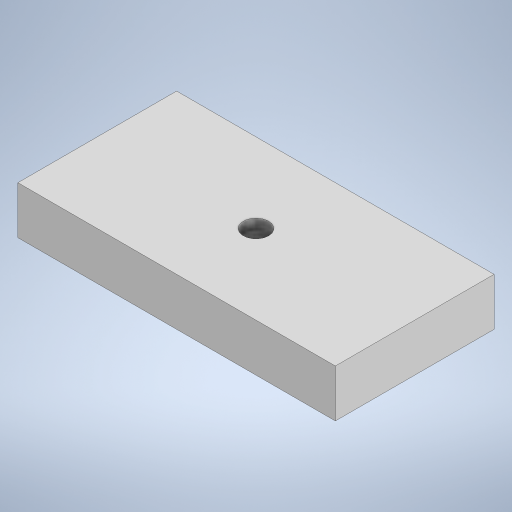
# Autodesk Inventor part: mocowanie osi
Saved by Autodesk Inventor 2024 (Build 280153000, 153)
## iProperties
Created: 2024-11-28
Part Number: mocowanie osi
Material: Ogólny
Document SubType Name: Modeling
Designer: fkoba.i_ekonomik
Density: 1 g/cm^3
Appearance: Domyślna
Author: fkoba.i_ekonomik
Autodesk Inventor part; units mm, degrees
ref_plane "YZ Plane" through (0, 0, 0) normal (1, 0, 0) x (0, 1, 0)
ref_plane "XZ Plane" through (0, 0, 0) normal (0, 1, 0) x (-1, 0, 0)
ref_plane "XY Plane" through (0, 0, 0) normal (0, 0, 1) x (1, 0, 0)
sketch "Szkic1" plane through (0, 0, 0) normal (0, 1, 0) x (-1, 0, 0)
  line L0 (100, -50) -> (-100, -50)
  line L1 (-100, -50) -> (-100, 50)
  line L2 (-100, 50) -> (100, 50)
  line L3 (100, 50) -> (100, -50)
  line L4 (140, 0) -> (-140, 0) projected
  line L5 (0, -70) -> (0, 70) projected
  point P0 (0, 0)
  dimension "d0" = 200
  dimension "d1" = 100
  constraints: 8 end point, 2 parallel, 1 horizontal, 1 perpendicular, 2 other
  measures "d0" distance of L0.start L0.end
  measures "d1" distance of L0.end L1.end
extrude "Wyciągnięcie proste1" add sketch "Szkic1" along normal blind 30
sketch "Szkic2" plane through (0, 30, 0) normal (0, 1, 0) x (1, 0, 0)
  point P0 (0, 0)
  point P1 (0, 0)
  constraints: 1 coincident
hole "Otwór1" at (0, 30, 0) direction (0, -1, 0) diameter 16 end through all
